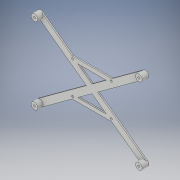
# Autodesk Inventor part: LCDv5-backCover
Saved by Autodesk Inventor 2018 (Build 220112000, 112)
## iProperties
Created: 2017-11-06
Part Number: LCDv5-backCover
Material: Generic
Document SubType Name: Modeling
Designer: WutchZone
Density: 1 g/cm^3
Appearance: Default
Author: WutchZone
Autodesk Inventor part; units mm, degrees
ref_plane "YZ Plane" through (0, 0, 0) normal (1, 0, 0) x (0, 1, 0)
ref_plane "XZ Plane" through (0, 0, 0) normal (0, 1, 0) x (-1, 0, 0)
ref_plane "XY Plane" through (0, 0, 0) normal (0, 0, 1) x (1, 0, 0)
sketch "Sketch1" plane through (0, 0, 0) normal (0, 0, 1) x (1, 0, 0)
  line L0 (92.45, -67.135) -> (-92.45, -67.135) construction
  line L1 (-92.45, -67.135) -> (-92.45, 67.135) construction
  line L2 (-92.45, 67.135) -> (92.45, 67.135) construction
  line L3 (92.45, 67.135) -> (92.45, -67.135) construction
  line L4 (92.45, -67.135) -> (-92.45, 67.135) construction
  line L5 (-92.45, -67.135) -> (92.45, 67.135) construction
  line L6 (77.45, -40.52) -> (-78.55, -40.52) construction
  line L7 (-78.55, -40.52) -> (-78.55, 48.48) construction
  line L8 (-78.55, 48.48) -> (77.45, 48.48) construction
  line L9 (77.45, 48.48) -> (77.45, -40.52) construction
  circle A0 centre (-78.45, 57.48) radius 1.5 construction
  circle A1 centre (-78.45, -57.48) radius 1.5 construction
  line L10 (0, 87.0056) -> (0, -123.2523) construction
  circle A2 centre (78.45, 57.48) radius 1.5 construction
  circle A3 centre (78.45, -57.48) radius 1.5 construction
  line L11 (-78.45, 57.48) -> (78.45, 57.48) construction
  line L12 (-78.45, 57.48) -> (-78.45, 67.135) construction
  line L13 (-78.45, -57.48) -> (-78.45, -67.135) construction
  circle A4 centre (-78.45, 57.48) radius 5
  circle A5 centre (78.45, 57.48) radius 5
  line L14 (-92.45, 0) -> (92.45, 0) construction
  circle A6 centre (-78.45, -57.48) radius 5
  circle A7 centre (78.45, -57.48) radius 5
  line L15 (-81.4051, 53.4467) -> (75.4949, -61.5133)
  line L16 (-75.4949, 61.5133) -> (81.4051, -53.4467)
  line L17 (-75.4949, -61.5133) -> (81.4051, 53.4467)
  line L18 (-81.4051, -53.4467) -> (75.4949, 61.5133)
  point P0 (0, 0)
  point P1 (0, 67.135)
  point P2 (-78.55, 3.98)
  point P3 (0, 57.48)
  dimension "d0" = 184.9
  dimension "d1" = 134.27
  dimension "d2" = 156
  dimension "d3" = 89
  dimension "d4" = 114.96
  dimension "d5" = 3
  dimension "d6" = 156.9
  dimension "d7" = 9
  dimension "d17" = 15
  dimension "d18" = 13.9
  dimension "d19" = 10
  constraints: 38 end point, 8 centre point, 8 point on circle, 8 tangent, 7 midpoint, 5 symmetric about line, 4 parallel, 4 perpendicular, 3 horizontal, 3 vertical alignment, 2 point on line, 1 coincident, 1 collinear, 1 equal radius, 1 vertical, 5 other
  measures "d0" distance of L1.end L2.end
  measures "d1" distance of L2.end L0.start
  measures "d2" distance of L7.end L8.end
  measures "d3" distance of L8.end L6.start
  measures "d4" distance of L13.start L11.start
  measures "d5" diameter of A0
  measures "d6" distance of L11.end L11.start
  measures "d7" distance from line of L11.start L8
  measures "d17" distance between parallel lines of L9 L3
  measures "d18" distance between parallel lines of L1 L7
  measures "d19" diameter of A4
extrude "Extrusion3" add sketch "Sketch1" against normal blind 2
sketch "Sketch3" plane through (0, 0, 0) normal (0, 0, 1) x (1, 0, 0)
  circle A0 centre (-78.45, 57.48) radius 5
  line L0 (0, 65.2064) -> (0, -49.8474) construction
  line L1 (-74.1059, 0) -> (81.0801, 0) construction
  arc A1 (-75.4949, 61.5133) -> (-81.4051, 53.4467) centre (-78.45, 57.48) ccw projected
  circle A2 centre (78.45, 57.48) radius 5
  circle A3 centre (-78.45, -57.48) radius 5
  circle A4 centre (78.45, -57.48) radius 5
  point P0 (0, 0)
  constraints: 4 centre point, 4 end point, 3 symmetric about line, 2 concentric, 2 point on line, 1 horizontal, 1 vertical, 3 other
extrude "Extrusion4" add sketch "Sketch3" along normal blind 8
sketch "Sketch4" plane through (-78.45, -57.48, 8) normal (0, 0, 1) x (1, 0, 0)
  circle A0 centre (0, 0) radius 1.55
  line L0 (-9.7734, 57.48) -> (187.2333, 57.48) construction
  line L1 (78.45, 128.3827) -> (78.45, -12.8511) construction
  circle A1 centre (156.9, 0) radius 1.55
  circle A2 centre (0, 114.96) radius 1.55
  circle A3 centre (156.9, 114.96) radius 1.55
  circle A4 centre (0, 0) radius 5 construction
  point P0 (78.45, 57.48)
  dimension "d24" = 3.1
  constraints: 4 centre point, 4 end point, 3 symmetric about line, 2 point on line, 1 concentric, 1 horizontal, 1 vertical, 3 other
  measures "d24" diameter of A0
extrude "Extrusion5" cut sketch "Sketch4" against normal up to next
sketch "Sketch5" plane through (0, 0, 0) normal (0, 0, 1) x (1, 0, 0)
  line L0 (-29, -24.5) -> (29, -24.5) construction
  line L1 (29, -24.5) -> (29, 24.5) construction
  line L2 (29, 24.5) -> (-29, 24.5) construction
  line L3 (-29, 24.5) -> (-29, -24.5) construction
  line L4 (-29, -24.5) -> (29, 24.5) construction
  line L5 (29, -24.5) -> (-29, 24.5) construction
  circle A0 centre (29, 24.5) radius 1.55
  line L6 (0, 47.6291) -> (0, -68.5673) construction
  line L7 (-80.197, 0) -> (59.821, 0) construction
  circle A1 centre (-29, 24.5) radius 1.55
  line L8 (29, -24.5) -> (-29, -24.5) construction
  circle A2 centre (29, -24.5) radius 1.55
  circle A3 centre (-29, -24.5) radius 1.55
  line L9 (0, 6.1985) -> (-75.4949, 61.5133) projected
  line L10 (-29.7552, 28) -> (29.7552, 28)
  line L11 (21.5663, 22) -> (-21.5663, 22)
  line L12 (75.4949, 61.5133) -> (0, 6.1985) projected
  line L13 (-29.7552, -28) -> (29.7552, -28)
  line L14 (21.5663, -22) -> (-21.5663, -22)
  line L15 (-29.7552, -28) -> (-21.5663, -22)
  line L16 (0, -6.1985) -> (-75.4949, -61.5133) projected
  line L17 (21.5663, -22) -> (29.7552, -28)
  line L18 (75.4949, -61.5133) -> (0, -6.1985) projected
  point P0 (0, 0)
  dimension "d27" = 58
  dimension "d28" = 49
  dimension "d29" = 3.1
  dimension "d30" = 6
  dimension "d31" = 2.5
  constraints: 30 end point, 7 symmetric about line, 4 centre point, 4 point on line, 3 coincident, 3 horizontal, 3 parallel, 2 collinear, 2 midpoint, 1 perpendicular, 1 vertical, 3 other
  measures "d27" distance of L1.end L2.end
  measures "d28" distance of L2.end L0.start
  measures "d29" diameter of A0
  measures "d30" distance between parallel lines of L11 L10
  measures "d31" distance between parallel lines of L2 L11
extrude "Extrusion6" add sketch "Sketch5" against normal up to surface (2 mm away) contours L9 L10 L12 L11 | L15 L14 L17 L13
extrude "Extrusion7" cut sketch "Sketch5" against normal up to next contours A0 | A1 | A2 | A3
body "Solid2"
